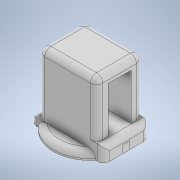
# Autodesk Inventor part: turret y
Saved by Autodesk Inventor 2020 (Build 240168000, 168)
## iProperties
Created: 2019-06-21
Part Number: turret y
Material: Generic
Document SubType Name: Modeling
Designer: kangh
Density: 1 g/cm^3
Appearance: Default
Author: kangh
Autodesk Inventor part; units mm, degrees
ref_plane "YZ Plane" through (0, 0, 0) normal (1, 0, 0) x (0, 1, 0)
ref_plane "XZ Plane" through (0, 0, 0) normal (0, 1, 0) x (-1, 0, 0)
ref_plane "XY Plane" through (0, 0, 0) normal (0, 0, 1) x (1, 0, 0)
sketch "Sketch1" plane through (0, 0, 0) normal (0, 1, 0) x (-1, 0, 0)
  circle A0 centre (0, 0) radius 19.05
  circle A1 centre (0, 0) radius 12.7
  circle A2 centre (0, 0) radius 4
  line L0 (12.7, 0) -> (11.2, 0)
  circle A3 centre (11.2, 0) radius 1.5
  line L1 (11.2, 1.5) -> (2.3814, 3.2139)
  line L2 (11.2, -1.5) -> (2.3814, -3.2139)
  circle A4 centre (0, 11.2) radius 1.5
  line L3 (-1.5, 11.2) -> (-3.2139, 2.3814)
  line L4 (1.5, 11.2) -> (3.2139, 2.3814)
  circle A5 centre (-11.2, 0) radius 1.5
  line L5 (-11.2, -1.5) -> (-2.3814, -3.2139)
  line L6 (-11.2, 1.5) -> (-2.3814, 3.2139)
  circle A6 centre (0, -11.2) radius 1.5
  line L7 (1.5, -11.2) -> (3.2139, -2.3814)
  line L8 (-1.5, -11.2) -> (-3.2139, -2.3814)
  point P0 (0, 12.7)
  point P1 (-12.7, 0)
  point P2 (0, -12.7)
  point P3 (3.0784, 3.0784)
  point P4 (3.0784, -3.0784)
  point P5 (-3.0784, -3.0784)
  point P6 (-3.0784, 3.0784)
  dimension "d1" = 25.4
  dimension "d0" = 38.1
  dimension "d2" = 8
  dimension "d3" = 1.5
  dimension "d6" = 360
  constraints: 18 end point, 14 point on circle, 6 centre point, 4 coincident, 1 horizontal, 1 horizontal alignment, 39 other
  measures "d0" diameter of A0
  measures "d2" diameter of A2
  measures "d3" distance of L0.start L0.end
extrude "Extrusion1" add sketch "Sketch1" along normal blind 2 contours A0 | A3 L1 L4 A4 A1 | A1 A6 L7 L2 A3 | A4 L3 L6 A5 A1 | A1 A5 L5 L8 A6
sketch "Sketch2" plane through (0, 2, 0) normal (0, 1, 0) x (1, 0, 0)
  circle A0 centre (0, 0) radius 19.05
  constraints: 1 centre point, 1 coincident
extrude "Extrusion2" add sketch "Sketch2" along normal blind 2
sketch "Sketch3" plane through (0, 4, 0) normal (0, 1, 0) x (1, 0, 0)
  circle A0 centre (0, 0) radius 19.05 projected
  line L0 (-19.05, 0) -> (-14.75, 0)
  line L1 (-14.75, 0) -> (-14.75, 12)
  line L2 (-14.75, 12) -> (-19.05, 12)
  line L3 (-19.05, 12) -> (-19.05, 0)
  line L4 (-19.05, 0) -> (-14.75, 0)
  line L5 (-14.75, 0) -> (-14.75, -12)
  line L6 (-14.75, -12) -> (-19.05, -12)
  line L7 (-19.05, -12) -> (-19.05, 0)
  line L8 (18.9689, 0) -> (14.6689, 0)
  line L9 (14.6689, 0) -> (14.6689, 12)
  line L10 (14.6689, 12) -> (18.9689, 12)
  line L11 (18.9689, 12) -> (18.9689, 0)
  line L12 (18.9689, 0) -> (14.6689, 0)
  line L13 (14.6689, 0) -> (14.6689, -12)
  line L14 (14.6689, -12) -> (18.9689, -12)
  line L15 (18.9689, -12) -> (18.9689, 0)
  dimension "d12" = 4.3
  dimension "d13" = 12
  dimension "d14" = 12
  dimension "d15" = 4.3
  constraints: 32 end point, 8 parallel, 5 point on line, 4 horizontal, 4 perpendicular, 1 horizontal alignment, 1 other
  measures "d12" distance of L2.end L1.end
  measures "d13" distance of L1.end L0.end
  measures "d14" distance of L4.end L5.end
  measures "d15" distance of L9.end L10.end
extrude "Extrusion3" add sketch "Sketch3" along normal mid plane 8 contours L11 L8 L9 L10 A0 | A0 L10 L11 | L15 L14 A0 | A0 L14 L13 L8 L15 | L2 L1 L0 A0 | A0 L3 L2 | L6 L7 A0 | A0 L0 L5 L6
sketch "Sketch4" plane through (-19.05, 0, 12) normal (-1, 0, 0) x (0, 0, 1)
  line L0 (0, 8) -> (-24, 8) projected
  line L1 (-12, 8) -> (-12, 32)
  line L2 (-12, 32) -> (-6, 32)
  line L3 (-12, 32) -> (-18, 32)
  line L4 (-18, 32) -> (-18, 8)
  line L5 (-6, 32) -> (-6, 8)
  line L6 (-18, 8) -> (-6, 8)
  line L7 (0, 4) -> (0, 8) projected
  line L8 (0, 8) -> (-24, 8)
  line L9 (-24, 8) -> (-24, 36.7561)
  line L10 (-24, 36.7561) -> (0, 36.7561)
  line L11 (0, 36.7561) -> (0, 8)
  point P0 (-12, 0)
  dimension "d18" = 24
  dimension "d19" = 6
  dimension "d20" = 6
  constraints: 20 end point, 3 horizontal, 3 perpendicular, 2 parallel, 2 point on line, 1 collinear, 1 midpoint, 1 vertical
  measures "d18" distance of L1.start L1.end
  measures "d19" distance of L1.end L2.end
  measures "d20" distance of L1.end L3.end
extrude "Extrusion4" add sketch "Sketch4" against normal blind 4.3 contours L0 L5 L2 L3 L4 L9 L10 L11
move faces "Move1" translate (30.1752, 0, 0) faces at (-14.75, 24.252, 10)
sketch "Sketch5" plane through (-19.05, 0, -12) normal (-1, 0, 0) x (0, 0, 1)
  line L0 (0, 4) -> (-7.05, 4) projected
  line L1 (0, 36.7561) -> (24, 36.7561) projected
  line L2 (0, 4) -> (24, 4)
  line L3 (24, 4) -> (24, 36.7561)
  line L4 (24, 36.7561) -> (0, 36.7561)
  line L5 (0, 36.7561) -> (0, 4)
  point P0 (12, 0)
  constraints: 8 end point, 2 parallel, 1 horizontal, 1 perpendicular
extrude "Extrusion5" cut sketch "Sketch5" against normal blind 4.3
fillet "Fillet1" radius 3.175 16 edges at (18.9689, 4, -12) (18.9689, 4, 12) (-19.05, 2, -12) (-19.05, 2, 12) (0.3376, 36.7561, -12) (0.3376, 36.7561, 12) (15.4252, 22.378, 12) (15.4252, 22.378, -12) (-14.75, 20.378, -12) (-14.75, 20.378, 12) (-14.75, 36.7561, 0) (15.4252, 36.7561, 0) (0, 4, -19.05) (-19.05, 4, 0) (0, 4, 19.05) (18.9689, 8, 0)
body "Solid1"
